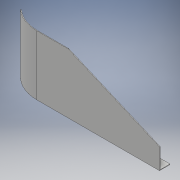
# Autodesk Inventor part: endplate_ver2
Saved by Autodesk Inventor 2018 (Build 220112000, 112)
## iProperties
Created: 2018-05-11
Part Number: endplate_ver2
Material: 一般
Document SubType Name: Modeling
Designer: ku_sk
Density: 1 g/cm^3
Appearance: 既定
Author: ku_sk
Autodesk Inventor part; units mm, degrees
ref_plane "YZ Plane" through (0, 0, 0) normal (1, 0, 0) x (0, 1, 0)
ref_plane "XZ Plane" through (0, 0, 0) normal (0, 1, 0) x (-1, 0, 0)
ref_plane "XY Plane" through (0, 0, 0) normal (0, 0, 1) x (1, 0, 0)
sketch "スケッチ1" plane through (0, 0, 0) normal (0, 1, 0) x (-1, 0, 0)
  line L0 (250, 100) -> (-250, 100)
  line L1 (-250, 100) -> (-250, -100)
  line L2 (-250, -100) -> (250, -100)
  line L3 (250, -100) -> (250, 100)
  point P0 (0, 0)
  dimension "d2" = 250
  dimension "d3" = 500
  dimension "d4" = 100
  dimension "d5" = 200
  constraints: 8 end point, 2 parallel, 1 horizontal, 1 perpendicular
  measures "d2" distance from line of point (0, 0) L3
  measures "d3" distance of L0.start L0.end
  measures "d4" distance from line of point (0, 0) L0
  measures "d5" distance of L2.end L0.start
extrude "押し出し1" add sketch "スケッチ1" along normal blind 35
sketch "スケッチ2" plane through (-250, 0, 100) normal (0, 0, 1) x (1, 0, 0)
  line L0 (0, 35) -> (500, 35) projected
  line L1 (0, 0) -> (500, 0) projected
  arc A0 (0, 35) -> (90, 0) centre (90, 133.2143) ccw
  line L2 (0, 0) -> (0, 35) projected
  point P0 (250, 0)
  dimension "d8" = 90
  constraints: 2 point on circle, 1 centre point, 1 point on line, 1 tangent
  measures "d8" distance from line of L2 A0.end
extrude "押し出し2" cut sketch "スケッチ2" against normal through all
shell "シェル1" thickness 2 removed faces 3 at (-53.3333, 23.3333, 100) at (250, 11.6667, 33.3333) at (83.3333, 35, 33.3333)
sketch "スケッチ3" plane through (0, 0, 0) normal (0, 1, 0) x (-1, 0, 0)
  line L0 (160, 100) -> (-250, 100) projected
  line L1 (55.6266, 100) -> (-250, -30.9191)
  line L2 (-250, 100) -> (-250, -100) projected
  point P0 (0, 0)
  constraints: 2 end point, 2 point on line
extrude "押し出し3" cut sketch "スケッチ3" along normal through all
